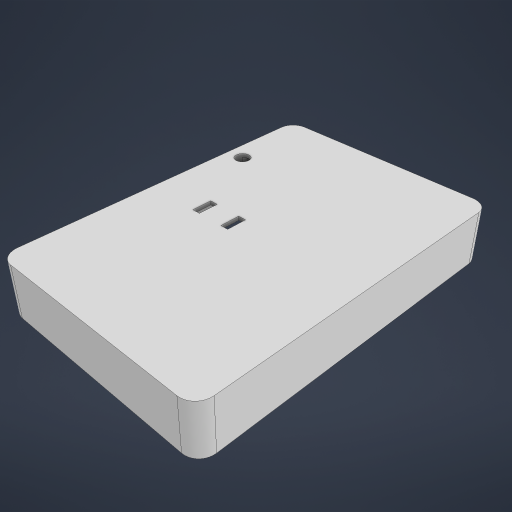
# Autodesk Inventor part: Pieza1
Saved by Autodesk Inventor 2023 (Build 270158000, 158)
## iProperties
Created: 2024-04-13
Part Number: Pieza1
Material: Genérico
Document SubType Name: Modeling
Designer: Diego
Density: 1 g/cm^3
Appearance: Valor por defecto
Author: Diego
Autodesk Inventor part; units mm, degrees
ref_plane "YZ Plane" through (0, 0, 0) normal (1, 0, 0) x (0, 1, 0)
ref_plane "XZ Plane" through (0, 0, 0) normal (0, 1, 0) x (-1, 0, 0)
ref_plane "XY Plane" through (0, 0, 0) normal (0, 0, 1) x (1, 0, 0)
sketch "Boceto1" plane through (0, 0, 0) normal (0, 1, 0) x (-1, 0, 0)
  line L0 (-25, 38) -> (25, 38)
  line L1 (25, 38) -> (25, -38)
  line L2 (25, -38) -> (-25, -38)
  line L3 (-25, -38) -> (-25, 38)
  line L4 (-25, 38) -> (25, -38) construction
  line L5 (25, 38) -> (-25, -38) construction
  line L6 (28, -37) -> (28, 37)
  line L7 (24, 41) -> (-24, 41)
  line L8 (-28, 37) -> (-28, -37)
  line L9 (-24, -41) -> (24, -41)
  arc A0 (28, 37) -> (24, 41) centre (24, 37) ccw
  arc A1 (24, -41) -> (28, -37) centre (24, -37) ccw
  arc A2 (-28, -37) -> (-24, -41) centre (-24, -37) ccw
  arc A3 (-24, 41) -> (-28, 37) centre (-24, 37) ccw
  point P0 (0, 0)
  dimension "d0" = 50
  dimension "d1" = 76
  dimension "d2" = 3
  dimension "d3" = 4
  constraints: 20 end point, 8 point on circle, 8 tangent, 4 centre point, 4 parallel, 3 equal radius, 2 midpoint, 2 perpendicular, 1 horizontal, 3 other
  measures "d0" distance of L1.end L2.end
  measures "d1" distance of L0.end L1.end
  measures "d2" distance between parallel lines of L1 L6
  measures "d3" radius of A0
extrude "Extrusión1" add sketch "Boceto1" along normal blind 12
sketch "Boceto2" plane through (0, 12, 0) normal (0, 1, 0) x (1, 0, 0)
  arc A0 (-28, -37) -> (-24, -41) centre (-24, -37) ccw projected
  line L0 (-24, -41) -> (24, -41) projected
  arc A1 (24, -41) -> (28, -37) centre (24, -37) ccw projected
  line L1 (28, -37) -> (28, 37) projected
  arc A2 (28, 37) -> (24, 41) centre (24, 37) ccw projected
  line L2 (24, 41) -> (-24, 41) projected
  arc A3 (-24, 41) -> (-28, 37) centre (-24, 37) ccw projected
  line L3 (-28, 37) -> (-28, -37) projected
  line L4 (25, -38) -> (-25, -38) projected
  line L5 (-25, -38) -> (-25, 38) projected
  line L6 (-25, 38) -> (25, 38) projected
  line L7 (25, 38) -> (25, -38) projected
  point P0 (0, 0)
extrude "Extrusión2" add sketch "Boceto2" along normal blind 1 contours L3 A3 L2 A2 L1 A1 L0 A0 | L4 L5 L6 L7
sketch "Boceto3" plane through (25, 0, -38) normal (-1, 0, 0) x (0, 0, 1)
  line L0 (0, 0) -> (76, 0) projected
  line L1 (76, 0) -> (76, 12) projected
  line L2 (0, 12) -> (76, 12) projected
  line L3 (0, 0) -> (0, 12) projected
  line L4 (5.5, 12) -> (13.5, 12)
  line L5 (15, 10.5) -> (15, 8)
  line L6 (13.5, 6.5) -> (5.5, 6.5)
  line L7 (4, 8) -> (4, 10.5)
  arc A0 (13.5, 6.5) -> (15, 8) centre (13.5, 8) ccw
  arc A1 (4, 8) -> (5.5, 6.5) centre (5.5, 8) ccw
  arc A2 (15, 10.5) -> (13.5, 12) centre (13.5, 10.5) ccw
  arc A3 (5.5, 12) -> (4, 10.5) centre (5.5, 10.5) ccw
  point P0 (38, 0)
  point P1 (15, 12)
  point P2 (15, 6.5)
  point P3 (4, 6.5)
  point P4 (4, 12)
  point P5 (13.5, 12)
  point P6 (5.5, 12)
  dimension "d8" = 15
  dimension "d9" = 5.5
  dimension "d10" = 11
  dimension "d11" = 90
  dimension "d12" = 5.5
  dimension "d13" = 90
  dimension "d14" = 1.5
  dimension "d15" = 1.5
  constraints: 9 point on line, 8 end point, 8 point on circle, 8 tangent, 4 centre point, 3 perpendicular, 2 equal radius
  measures "d8" distance of L2.start point (15, 12)
  measures "d9" distance of point (15, 12) point (15, 6.5)
  measures "d10" distance of point (15, 6.5) point (4, 6.5)
  measures "d11" angle of L5 L6
  measures "d12" distance of point (4, 6.5) point (4, 12)
  measures "d13" angle of L6 L7
  measures "d14" radius of A0
  measures "d15" radius of A2
extrude "Extrusión3" cut sketch "Boceto3" along normal through all contours L2 A2 L5 A0 L6 A1 L7 A3
sketch "Boceto4" plane through (-25, 0, -38) normal (0, 0, 1) x (1, 0, 0)
  line L0 (0, 0) -> (50, 0) projected
  line L1 (50, 0) -> (50, 12) projected
  line L2 (0, 12) -> (50, 12) projected
  line L3 (0, 0) -> (0, 12) projected
  line L4 (0, 12) -> (25.5, 12)
  line L5 (25.5, 12) -> (25.5, 4.5)
  line L6 (25.5, 4.5) -> (12, 4.5)
  line L7 (25.5, 12) -> (25.5, 8.5)
  line L8 (25.5, 8.5) -> (12, 8.5)
  line L9 (12, 8.5) -> (12, 4.5)
  point P0 (25, 0)
  dimension "d18" = 25.5
  dimension "d19" = 7.5
  dimension "d20" = 13.5
  dimension "d21" = 3.5
  constraints: 12 end point, 4 perpendicular, 2 point on line
  measures "d18" distance of L2.start L4.end
  measures "d19" distance of L4.end L5.end
  measures "d20" distance of L5.end L6.end
  measures "d21" distance of L4.end L7.end
extrude "Extrusión4" cut sketch "Boceto4" against normal blind 10 contours L5 L6 L9 L8
sketch "Boceto5" plane through (0, 12, 0) normal (0, -1, 0) x (1, 0, 0)
  line L0 (-25, -32.5) -> (-25, -38) projected
  line L1 (-25, -38) -> (25, -38) projected
  line L2 (25, -38) -> (25, 38) projected
  line L3 (25, 38) -> (-25, 38) projected
  line L4 (-25, 38) -> (-25, -24.5) projected
  line L5 (-25, -24.5) -> (-28, -24.5) projected
  line L6 (-28, -32.5) -> (-28, -24.5) projected
  line L7 (-25, -32.5) -> (-28, -32.5) projected
  line L8 (-25, -23) -> (-25, -24.5) projected
  line L9 (-25, 38) -> (-25, -24.5) projected
  line L10 (-25, 38) -> (-25, -38) projected
  line L11 (-25, -32.5) -> (-25, -38) projected
  line L12 (-25, -32.5) -> (-25, -34) projected
  line L13 (-25, -34) -> (-25, -32.5) projected
  line L14 (-25, -32.5) -> (-25, -24.5) projected
  line L15 (-25, -24.5) -> (-25, -23) projected
  line L16 (-25, -23) -> (-25, -19.1)
  line L17 (-25, -23) -> (-21.1, -23) construction
  line L18 (-25, -19.1) -> (-23.5, -19.1)
  circle A0 centre (-23.5, -19.1) radius 2
  point P0 (0, 0)
  dimension "d24" = 3.9
  dimension "d25" = 90
  dimension "d26" = 1.5
  dimension "d27" = 4
  constraints: 6 end point, 2 perpendicular, 1 centre point, 1 coincident, 1 collinear, 1 horizontal
  measures "d24" distance of L15.end L16.end
  measures "d25" angle of L17 L16
  measures "d26" distance of L16.end L18.end
  measures "d27" diameter of A0
extrude "Extrusión5" cut sketch "Boceto5" along normal mid plane 14 contours A0 L4 | L4 A0
sketch "Boceto6" plane through (0, 12, 0) normal (0, -1, 0) x (1, 0, 0)
  arc A0 (-25, -20.4229) -> (-25, -17.7771) centre (-23.5, -19.1) ccw projected
  line L0 (-25, -20.4229) -> (-25, -24.5) projected
  line L1 (-25, -24.5) -> (-28, -24.5) projected
  line L2 (-28, -32.5) -> (-28, -24.5) projected
  line L3 (-25, -32.5) -> (-28, -32.5) projected
  line L4 (-25, -32.5) -> (-25, -38) projected
  line L5 (-25, -38) -> (25, -38) projected
  line L6 (25, -38) -> (25, 38) projected
  line L7 (25, 38) -> (-25, 38) projected
  line L8 (-25, 38) -> (-25, -17.7771) projected
  line L9 (-6, 4) -> (-4, 4)
  line L10 (-4, 4) -> (-4, -1)
  line L11 (-4, -1) -> (-6, -1)
  line L12 (-6, -1) -> (-6, 4)
  line L13 (-6, 4) -> (-4, -1) construction
  line L14 (-4, 4) -> (-6, -1) construction
  line L15 (-14.5, 4) -> (-12.5, 4)
  line L16 (-12.5, 4) -> (-12.5, -1)
  line L17 (-12.5, -1) -> (-14.5, -1)
  line L18 (-14.5, -1) -> (-14.5, 4)
  line L19 (-14.5, 4) -> (-12.5, -1) construction
  line L20 (-12.5, 4) -> (-14.5, -1) construction
  point P0 (0, 0)
  point P1 (-13.5, 1.5)
  point P2 (-5, 1.5)
  dimension "d30" = 11.5
  dimension "d31" = 39.5
  dimension "d32" = 8.5
  dimension "d33" = 2
  dimension "d34" = 5
  dimension "d35" = 2
  dimension "d36" = 5
  constraints: 24 end point, 4 midpoint, 4 parallel, 2 horizontal, 2 perpendicular
  measures "d30" distance from line of L8 point (-13.5, 1.5)
  measures "d31" distance from line of L5 point (-13.5, 1.5)
  measures "d32" distance of point (-5, 1.5) point (-13.5, 1.5)
  measures "d33" distance of L10.end L11.end
  measures "d34" distance of L9.end L10.end
  measures "d35" distance of L16.end L17.end
  measures "d36" distance of L15.end L16.end
extrude "Extrusión6" cut sketch "Boceto6" against normal blind 14 contours L9 L10 L11 L12 | L15 L16 L17 L18
